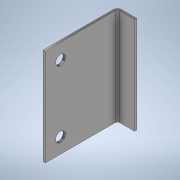
# Autodesk Inventor part: Sujeta Porta Suero-sin tubo
Saved by Autodesk Inventor 2020.3 (Build 243373000, 373)
## iProperties
Created: 2020-06-30
Part Number: Sujeta Porta Suero-sin tubo
Material: Steel, Carbon
Document SubType Name: Sheet Metal
Designer: Bruno
Density: 7.85 g/cm^3
Sheet Metal Rule: Default_mm
Appearance: Semi-Polished
Author: Bruno
Autodesk Inventor part; units mm, degrees
ref_plane "YZ Plane" through (0, 0, 0) normal (1, 0, 0) x (0, 1, 0)
ref_plane "XZ Plane" through (0, 0, 0) normal (0, 1, 0) x (-1, 0, 0)
ref_plane "XY Plane" through (0, 0, 0) normal (0, 0, 1) x (1, 0, 0)
sketch "Sketch1" plane through (0, 0, 0) normal (1, 0, 0) x (0, 1, 0)
  line L0 (0, 0) -> (45, 0)
  line L1 (45, 0) -> (45, -34.5)
  line L2 (45, -34.5) -> (0, -34.5)
  line L3 (0, -34.5) -> (0, 0)
  dimension "d0" = 45
  dimension "d1" = 34.5
  measures "d0" distance of L1.end L2.end
  measures "d1" distance of L0.end L1.end
extrude "Plate1" add sketch "Sketch1" along normal blind 1
sketch "Sketch2" plane through (0, 45, -33.5) normal (0, 0, -1) x (-1, 0, 0)
  line L0 (0, -45) -> (0, 0)
  line L1 (0, 0) -> (-9, 0)
  line L2 (-9, 0) -> (-9, -45)
  line L3 (-9, -45) -> (0, -45)
  constraints: 6 end point, 1 horizontal, 1 perpendicular, 1 vertical
edge flange "Flange1" height 9 angle 90 thickness 1 bend radius 1 thickness toward (0, 0, -1) relief straight relief width 1 relief depth 0.5 edges at (1, 22.5, -34.5) wall of the first edge with corners at (0, 0, -33.5) (0, 45, -33.5) (9, 45, -33.5) (9, 0, -33.5)
bend "Bend1"
corner "Corner1"
sketch "Sketch3" plane through (1, 0, 0) normal (1, 0, 0) x (0, 0, -1)
  line L0 (0, 45) -> (32.5, 45) projected
  line L1 (0, 0) -> (0, 45) projected
  line L2 (32.5, 0) -> (0, 0) projected
  point P0 (7, 38)
  point P1 (7, 7)
  dimension "d13" = 7
  dimension "d14" = 7
  dimension "d15" = 7
  constraints: 1 vertical alignment
  measures "d13" distance from line of L0 point (7, 38)
  measures "d14" distance from line of L1 point (7, 38)
  measures "d15" distance from line of L2 point (7, 7)
hole "Hole1" at (1, 38, -7) at (1, 7, -7) direction (-1, 0, 0) diameter 4.5 end through all
equation "\"d15\" = d13"
equation "\"d21\" = Thickness"
equation "\"d2\" = Thickness"
equation "\"d3\" = BendReliefWidth"
equation "\"d4\" = BendReliefDepth"
equation "\"d5\" = MinimumRemnant"
equation "\"d6\" = TransitionRadius"
equation "\"d9\" = BendRadius"
equation "\"d10\" = CornerReliefSize"
equation "\"d11\" = GapSize"
equation "\"d12\" = JacobiRadiusSize"
equation "\"BendRadius\" = Thickness"
equation "\"BendReliefWidth\" = Thickness"
equation "\"BendReliefDepth\" = 0.5 * Thickness"
equation "\"CornerReliefSize\" = 4 * Thickness"
equation "\"MinimumRemnant\" = 2 * Thickness"
equation "\"TransitionRadius\" = BendRadius"
equation "\"JacobiRadiusSize\" = BendRadius"
equation "\"GapSize\" = Thickness"
equation "\"Thickness\" = 1"
body "Solid1"
